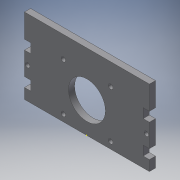
# Autodesk Inventor part: Motor_brace_2
Saved by Autodesk Inventor 2019 (Build 230136000, 136)
## iProperties
Created: 2020-03-11
Part Number: Motor_brace_2
Material: Generic
Document SubType Name: Modeling
Designer: Vijay
Density: 1 g/cm^3
Appearance: Default
Author: Vijay
Autodesk Inventor part; units mm, degrees
ref_plane "YZ Plane" through (0, 0, 0) normal (1, 0, 0) x (0, 1, 0)
ref_plane "XZ Plane" through (0, 0, 0) normal (0, 1, 0) x (-1, 0, 0)
ref_plane "XY Plane" through (0, 0, 0) normal (0, 0, 1) x (1, 0, 0)
sketch "Sketch1" plane through (0, 0, 0) normal (0, 0, 1) x (1, 0, 0)
  line L0 (20, 35.0868) -> (15.0858, 40.001) construction
  line L1 (15.0858, 40.001) -> (-15.0858, 40.001) construction
  line L2 (-15.0858, 40.001) -> (-20, 35.0868) construction
  line L3 (-20, 35.0868) -> (-20, 4.9152) construction
  line L4 (-20, 4.9152) -> (-15.0858, 0.001) construction
  line L5 (-15.0858, 0.001) -> (15.0858, 0.001) construction
  line L6 (15.0858, 0.001) -> (20, 4.9152) construction
  line L7 (20, 4.9152) -> (20, 35.0868) construction
  spline S0 degree 3 poles (-17.5, 4.501) (-17.5, 4.4448) (-17.4976, 4.3891) (-17.4883, 4.2777) (-17.4812, 4.2221) (-17.4625, 4.1117) (-17.4509, 4.0569) (-17.423, 3.9488) (-17.4069, 3.8953) (-17.3846, 3.8313) (-17.3806, 3.8202) (-17.3733, 3.8003) (-17.3701, 3.792) (-17.3645, 3.7774) (-17.3621, 3.7713) (-17.3394, 3.714) (-17.3174, 3.6644) (-17.2693, 3.567) (-17.2432, 3.5192) (-17.1873, 3.4259) (-17.1575, 3.3805) (-17.0943, 3.2923) (-17.061, 3.2495) (-16.9905, 3.1663) (-16.9533, 3.1259) (-16.8745, 3.0471) (-16.8335, 3.0095) (-16.7483, 2.9374) (-16.704, 2.9031) (-16.6129, 2.8383) (-16.566, 2.8079) (-16.4701, 2.7511) (-16.4211, 2.7248) (-16.3422, 2.6867) (-16.3133, 2.6735) (-16.2744, 2.657) (-16.2645, 2.6528) (-16.2484, 2.6463) (-16.2421, 2.6438) (-16.1856, 2.6214) (-16.1347, 2.6037) (-16.0314, 2.5722) (-15.979, 2.5585) (-15.8734, 2.5355) (-15.8202, 2.5261) (-15.7135, 2.5117) (-15.66, 2.5067) (-15.5709, 2.502) (-15.5355, 2.501) (-15.4438, 2.501) (-15.3881, 2.5034) (-15.2767, 2.5127) (-15.2211, 2.5198) (-15.1106, 2.5385) (-15.0559, 2.5501) (-14.9477, 2.578) (-14.8942, 2.5941) (-14.8302, 2.6164) (-14.8192, 2.6204) (-14.7993, 2.6277) (-14.791, 2.6309) (-14.7764, 2.6365) (-14.7703, 2.6389) (-14.713, 2.6616) (-14.6634, 2.6836) (-14.566, 2.7317) (-14.5182, 2.7578) (-14.4249, 2.8137) (-14.3795, 2.8435) (-14.2913, 2.9067) (-14.2485, 2.94) (-14.1653, 3.0105) (-14.1249, 3.0477) (-14.0461, 3.1265) (-14.0085, 3.1675) (-13.9364, 3.2527) (-13.9021, 3.297) (-13.8373, 3.3881) (-13.8069, 3.435) (-13.7501, 3.5309) (-13.7238, 3.5799) (-13.6857, 3.6588) (-13.6725, 3.6877) (-13.656, 3.7265) (-13.6519, 3.7364) (-13.6453, 3.7525) (-13.6428, 3.7589) (-13.6197, 3.8172) (-13.6014, 3.87) (-13.569, 3.9772) (-13.5551, 4.0317) (-13.5319, 4.1414) (-13.5226, 4.1967) (-13.5087, 4.3076) (-13.504, 4.3632) (-13.5006, 4.4464) (-13.5, 4.4736) (-13.5, 4.501) knots 0.5 0.5 0.5 0.5 0.513789 0.513789 0.527784 0.527784 0.541793 0.541793 0.555687 0.555687 0.558594 0.558594 0.560925 0.560925 0.5625 0.5625 0.574861 0.574861 0.587418 0.587418 0.599984 0.599984 0.612492 0.612492 0.625 0.625 0.637686 0.637686 0.650587 0.650587 0.663509 0.663509 0.676325 0.676325 0.683594 0.683594 0.68594 0.68594 0.6875 0.6875 0.700841 0.700841 0.714366 0.714366 0.727891 0.727891 0.741278 0.741278 0.75 0.75 0.76379 0.76379 0.777788 0.777788 0.7918 0.7918 0.805696 0.805696 0.808594 0.808594 0.810925 0.810925 0.8125 0.8125 0.824861 0.824861 0.837418 0.837418 0.849984 0.849984 0.862492 0.862492 0.875 0.875 0.887686 0.887686 0.900587 0.900587 0.913509 0.913509 0.926325 0.926325 0.933594 0.933594 0.935925 0.935925 0.9375 0.9375 0.951347 0.951347 0.96538 0.96538 0.979408 0.979408 0.993282 0.993282 1 1 1 1 construction
  spline S1 degree 3 poles (-13.5, 4.501) (-13.5, 4.5571) (-13.5024, 4.6127) (-13.5117, 4.7238) (-13.5187, 4.7793) (-13.5373, 4.8895) (-13.5489, 4.9441) (-13.5766, 5.0521) (-13.5927, 5.1054) (-13.6151, 5.1697) (-13.6192, 5.1812) (-13.6267, 5.2016) (-13.6299, 5.2101) (-13.6355, 5.2247) (-13.6379, 5.2308) (-13.6606, 5.288) (-13.6826, 5.3376) (-13.7307, 5.435) (-13.7568, 5.4828) (-13.8127, 5.5761) (-13.8425, 5.6215) (-13.9057, 5.7097) (-13.939, 5.7525) (-14.0095, 5.8357) (-14.0467, 5.8761) (-14.1255, 5.9549) (-14.1665, 5.9925) (-14.2517, 6.0646) (-14.296, 6.0989) (-14.3871, 6.1637) (-14.434, 6.1941) (-14.5299, 6.2509) (-14.5789, 6.2772) (-14.6578, 6.3153) (-14.6867, 6.3285) (-14.7256, 6.345) (-14.7355, 6.3492) (-14.7516, 6.3557) (-14.7579, 6.3582) (-14.8144, 6.3806) (-14.8653, 6.3983) (-14.9686, 6.4298) (-15.021, 6.4435) (-15.1266, 6.4665) (-15.1798, 6.4759) (-15.2865, 6.4903) (-15.34, 6.4953) (-15.4291, 6.5) (-15.4645, 6.501) (-15.5562, 6.501) (-15.6119, 6.4986) (-15.7233, 6.4893) (-15.7789, 6.4822) (-15.8894, 6.4635) (-15.9441, 6.4519) (-16.0523, 6.424) (-16.1058, 6.4079) (-16.1698, 6.3856) (-16.1808, 6.3816) (-16.2007, 6.3743) (-16.209, 6.3711) (-16.2236, 6.3655) (-16.2297, 6.3631) (-16.287, 6.3404) (-16.3366, 6.3184) (-16.434, 6.2703) (-16.4818, 6.2442) (-16.5751, 6.1883) (-16.6205, 6.1585) (-16.7087, 6.0953) (-16.7515, 6.062) (-16.8347, 5.9915) (-16.8751, 5.9543) (-16.9539, 5.8755) (-16.9915, 5.8345) (-17.0636, 5.7493) (-17.0979, 5.705) (-17.1627, 5.6139) (-17.1931, 5.567) (-17.2499, 5.4711) (-17.2762, 5.4221) (-17.3143, 5.3432) (-17.3275, 5.3143) (-17.344, 5.2754) (-17.3482, 5.2655) (-17.3547, 5.2494) (-17.3572, 5.2431) (-17.3796, 5.1866) (-17.3973, 5.1357) (-17.4288, 5.0324) (-17.4425, 4.98) (-17.4655, 4.8745) (-17.4749, 4.8213) (-17.4893, 4.7146) (-17.4943, 4.6611) (-17.4991, 4.5719) (-17.5, 4.5366) (-17.5, 4.501) knots 0 0 0 0 0.013787 0.013787 0.027761 0.027761 0.041736 0.041736 0.055579 0.055579 0.058594 0.058594 0.060939 0.060939 0.0625 0.0625 0.074861 0.074861 0.087418 0.087418 0.099984 0.099984 0.112492 0.112492 0.125 0.125 0.137686 0.137686 0.150587 0.150587 0.163509 0.163509 0.176325 0.176325 0.183594 0.183594 0.18594 0.18594 0.1875 0.1875 0.200841 0.200841 0.214366 0.214366 0.227891 0.227891 0.241278 0.241278 0.25 0.25 0.26379 0.26379 0.277788 0.277788 0.2918 0.2918 0.305696 0.305696 0.308594 0.308594 0.310925 0.310925 0.3125 0.3125 0.324861 0.324861 0.337418 0.337418 0.349984 0.349984 0.362492 0.362492 0.375 0.375 0.387686 0.387686 0.400587 0.400587 0.413509 0.413509 0.426325 0.426325 0.433594 0.433594 0.43594 0.43594 0.4375 0.4375 0.450839 0.450839 0.464362 0.464362 0.477886 0.477886 0.49127 0.49127 0.5 0.5 0.5 0.5 construction
  spline S2 degree 3 poles (-17.5, 35.501) (-17.5, 35.4448) (-17.4976, 35.3891) (-17.4883, 35.2777) (-17.4812, 35.2221) (-17.4625, 35.1117) (-17.4509, 35.0569) (-17.423, 34.9488) (-17.4069, 34.8953) (-17.3846, 34.8313) (-17.3806, 34.8202) (-17.3733, 34.8003) (-17.3701, 34.792) (-17.3645, 34.7774) (-17.3621, 34.7713) (-17.3394, 34.714) (-17.3174, 34.6644) (-17.2693, 34.567) (-17.2432, 34.5192) (-17.1873, 34.4259) (-17.1575, 34.3805) (-17.0943, 34.2923) (-17.061, 34.2495) (-16.9905, 34.1663) (-16.9533, 34.1259) (-16.8745, 34.0471) (-16.8335, 34.0095) (-16.7483, 33.9374) (-16.704, 33.9031) (-16.6129, 33.8383) (-16.566, 33.8079) (-16.4701, 33.7511) (-16.4211, 33.7248) (-16.3422, 33.6867) (-16.3133, 33.6735) (-16.2744, 33.657) (-16.2645, 33.6528) (-16.2484, 33.6463) (-16.2421, 33.6438) (-16.1856, 33.6214) (-16.1347, 33.6037) (-16.0314, 33.5722) (-15.979, 33.5585) (-15.8734, 33.5355) (-15.8202, 33.5261) (-15.7135, 33.5117) (-15.66, 33.5067) (-15.5709, 33.502) (-15.5355, 33.501) (-15.4438, 33.501) (-15.3881, 33.5034) (-15.2767, 33.5127) (-15.2211, 33.5198) (-15.1106, 33.5385) (-15.0559, 33.5501) (-14.9477, 33.578) (-14.8942, 33.5941) (-14.8302, 33.6164) (-14.8192, 33.6204) (-14.7993, 33.6277) (-14.791, 33.6309) (-14.7764, 33.6365) (-14.7703, 33.6389) (-14.713, 33.6616) (-14.6634, 33.6836) (-14.566, 33.7317) (-14.5182, 33.7578) (-14.4249, 33.8137) (-14.3795, 33.8435) (-14.2913, 33.9067) (-14.2485, 33.94) (-14.1653, 34.0105) (-14.1249, 34.0477) (-14.0461, 34.1265) (-14.0085, 34.1675) (-13.9364, 34.2527) (-13.9021, 34.297) (-13.8373, 34.3881) (-13.8069, 34.435) (-13.7501, 34.5309) (-13.7238, 34.5799) (-13.6857, 34.6588) (-13.6725, 34.6877) (-13.656, 34.7265) (-13.6519, 34.7364) (-13.6453, 34.7525) (-13.6428, 34.7589) (-13.6197, 34.8172) (-13.6014, 34.87) (-13.569, 34.9772) (-13.5551, 35.0317) (-13.5319, 35.1414) (-13.5226, 35.1967) (-13.5087, 35.3076) (-13.504, 35.3632) (-13.5006, 35.4464) (-13.5, 35.4736) (-13.5, 35.501) knots 0.5 0.5 0.5 0.5 0.513789 0.513789 0.527784 0.527784 0.541793 0.541793 0.555687 0.555687 0.558594 0.558594 0.560925 0.560925 0.5625 0.5625 0.574861 0.574861 0.587418 0.587418 0.599984 0.599984 0.612492 0.612492 0.625 0.625 0.637686 0.637686 0.650587 0.650587 0.663509 0.663509 0.676325 0.676325 0.683594 0.683594 0.68594 0.68594 0.6875 0.6875 0.700841 0.700841 0.714366 0.714366 0.727891 0.727891 0.741278 0.741278 0.75 0.75 0.76379 0.76379 0.777788 0.777788 0.7918 0.7918 0.805696 0.805696 0.808594 0.808594 0.810925 0.810925 0.8125 0.8125 0.824861 0.824861 0.837418 0.837418 0.849984 0.849984 0.862492 0.862492 0.875 0.875 0.887686 0.887686 0.900587 0.900587 0.913509 0.913509 0.926325 0.926325 0.933594 0.933594 0.935925 0.935925 0.9375 0.9375 0.951347 0.951347 0.96538 0.96538 0.979408 0.979408 0.993282 0.993282 1 1 1 1 construction
  spline S3 degree 3 poles (-13.5, 35.501) (-13.5, 35.5571) (-13.5024, 35.6127) (-13.5117, 35.7238) (-13.5187, 35.7793) (-13.5373, 35.8895) (-13.5489, 35.9441) (-13.5766, 36.0521) (-13.5927, 36.1054) (-13.6151, 36.1697) (-13.6192, 36.1812) (-13.6267, 36.2016) (-13.6299, 36.2101) (-13.6355, 36.2247) (-13.6379, 36.2308) (-13.6606, 36.288) (-13.6826, 36.3376) (-13.7307, 36.435) (-13.7568, 36.4828) (-13.8127, 36.5761) (-13.8425, 36.6215) (-13.9057, 36.7097) (-13.939, 36.7525) (-14.0095, 36.8357) (-14.0467, 36.8761) (-14.1255, 36.9549) (-14.1665, 36.9925) (-14.2517, 37.0646) (-14.296, 37.0989) (-14.3871, 37.1637) (-14.434, 37.1941) (-14.5299, 37.2509) (-14.5789, 37.2772) (-14.6578, 37.3153) (-14.6867, 37.3285) (-14.7256, 37.345) (-14.7355, 37.3492) (-14.7516, 37.3557) (-14.7579, 37.3582) (-14.8144, 37.3806) (-14.8653, 37.3983) (-14.9686, 37.4298) (-15.021, 37.4435) (-15.1266, 37.4665) (-15.1798, 37.4759) (-15.2865, 37.4903) (-15.34, 37.4953) (-15.4291, 37.5) (-15.4645, 37.501) (-15.5562, 37.501) (-15.6119, 37.4986) (-15.7233, 37.4893) (-15.7789, 37.4822) (-15.8894, 37.4635) (-15.9441, 37.4519) (-16.0523, 37.424) (-16.1058, 37.4079) (-16.1698, 37.3856) (-16.1808, 37.3816) (-16.2007, 37.3743) (-16.209, 37.3711) (-16.2236, 37.3655) (-16.2297, 37.3631) (-16.287, 37.3404) (-16.3366, 37.3184) (-16.434, 37.2703) (-16.4818, 37.2442) (-16.5751, 37.1883) (-16.6205, 37.1585) (-16.7087, 37.0953) (-16.7515, 37.062) (-16.8347, 36.9915) (-16.8751, 36.9543) (-16.9539, 36.8755) (-16.9915, 36.8345) (-17.0636, 36.7493) (-17.0979, 36.705) (-17.1627, 36.6139) (-17.1931, 36.567) (-17.2499, 36.4711) (-17.2762, 36.4221) (-17.3143, 36.3432) (-17.3275, 36.3143) (-17.344, 36.2754) (-17.3482, 36.2655) (-17.3547, 36.2494) (-17.3572, 36.2431) (-17.3796, 36.1866) (-17.3973, 36.1357) (-17.4288, 36.0324) (-17.4425, 35.98) (-17.4655, 35.8745) (-17.4749, 35.8213) (-17.4893, 35.7146) (-17.4943, 35.6611) (-17.4991, 35.5719) (-17.5, 35.5366) (-17.5, 35.501) knots 0 0 0 0 0.013787 0.013787 0.027761 0.027761 0.041736 0.041736 0.055579 0.055579 0.058594 0.058594 0.060939 0.060939 0.0625 0.0625 0.074861 0.074861 0.087418 0.087418 0.099984 0.099984 0.112492 0.112492 0.125 0.125 0.137686 0.137686 0.150587 0.150587 0.163509 0.163509 0.176325 0.176325 0.183594 0.183594 0.18594 0.18594 0.1875 0.1875 0.200841 0.200841 0.214366 0.214366 0.227891 0.227891 0.241278 0.241278 0.25 0.25 0.26379 0.26379 0.277788 0.277788 0.2918 0.2918 0.305696 0.305696 0.308594 0.308594 0.310925 0.310925 0.3125 0.3125 0.324861 0.324861 0.337418 0.337418 0.349984 0.349984 0.362492 0.362492 0.375 0.375 0.387686 0.387686 0.400587 0.400587 0.413509 0.413509 0.426325 0.426325 0.433594 0.433594 0.43594 0.43594 0.4375 0.4375 0.450839 0.450839 0.464362 0.464362 0.477886 0.477886 0.49127 0.49127 0.5 0.5 0.5 0.5 construction
  circle A0 centre (0, 20.001) radius 11 construction
  spline S4 degree 3 poles (13.5, 35.501) (13.5, 35.4448) (13.5024, 35.3891) (13.5117, 35.2777) (13.5188, 35.2221) (13.5375, 35.1117) (13.5491, 35.0569) (13.577, 34.9488) (13.5931, 34.8953) (13.6154, 34.8313) (13.6194, 34.8202) (13.6267, 34.8003) (13.6299, 34.792) (13.6355, 34.7774) (13.6379, 34.7713) (13.6606, 34.714) (13.6826, 34.6644) (13.7307, 34.567) (13.7568, 34.5192) (13.8127, 34.4259) (13.8425, 34.3805) (13.9057, 34.2923) (13.939, 34.2495) (14.0095, 34.1663) (14.0467, 34.1259) (14.1255, 34.0471) (14.1665, 34.0095) (14.2517, 33.9374) (14.296, 33.9031) (14.3871, 33.8383) (14.434, 33.8079) (14.5299, 33.7511) (14.5789, 33.7248) (14.6578, 33.6867) (14.6867, 33.6735) (14.7256, 33.657) (14.7355, 33.6528) (14.7516, 33.6463) (14.7579, 33.6438) (14.8144, 33.6214) (14.8653, 33.6037) (14.9686, 33.5722) (15.021, 33.5585) (15.1266, 33.5355) (15.1798, 33.5261) (15.2865, 33.5117) (15.34, 33.5067) (15.4291, 33.502) (15.4645, 33.501) (15.5562, 33.501) (15.6119, 33.5034) (15.7233, 33.5127) (15.7789, 33.5198) (15.8894, 33.5385) (15.9441, 33.5501) (16.0523, 33.578) (16.1058, 33.5941) (16.1698, 33.6164) (16.1808, 33.6204) (16.2007, 33.6277) (16.209, 33.6309) (16.2236, 33.6365) (16.2297, 33.6389) (16.287, 33.6616) (16.3366, 33.6836) (16.434, 33.7317) (16.4818, 33.7578) (16.5751, 33.8137) (16.6205, 33.8435) (16.7087, 33.9067) (16.7515, 33.94) (16.8347, 34.0105) (16.8751, 34.0477) (16.9539, 34.1265) (16.9915, 34.1675) (17.0636, 34.2527) (17.0979, 34.297) (17.1627, 34.3881) (17.1931, 34.435) (17.2499, 34.5309) (17.2762, 34.5799) (17.3143, 34.6588) (17.3275, 34.6877) (17.344, 34.7265) (17.3481, 34.7364) (17.3547, 34.7525) (17.3572, 34.7589) (17.3803, 34.8172) (17.3986, 34.87) (17.431, 34.9772) (17.4449, 35.0317) (17.4681, 35.1414) (17.4774, 35.1967) (17.4913, 35.3076) (17.496, 35.3632) (17.4994, 35.4464) (17.5, 35.4736) (17.5, 35.501) knots 0.5 0.5 0.5 0.5 0.513789 0.513789 0.527784 0.527784 0.541793 0.541793 0.555687 0.555687 0.558594 0.558594 0.560925 0.560925 0.5625 0.5625 0.574861 0.574861 0.587418 0.587418 0.599984 0.599984 0.612492 0.612492 0.625 0.625 0.637686 0.637686 0.650587 0.650587 0.663509 0.663509 0.676325 0.676325 0.683594 0.683594 0.68594 0.68594 0.6875 0.6875 0.700841 0.700841 0.714366 0.714366 0.727891 0.727891 0.741278 0.741278 0.75 0.75 0.76379 0.76379 0.777788 0.777788 0.7918 0.7918 0.805696 0.805696 0.808594 0.808594 0.810925 0.810925 0.8125 0.8125 0.824861 0.824861 0.837418 0.837418 0.849984 0.849984 0.862492 0.862492 0.875 0.875 0.887686 0.887686 0.900587 0.900587 0.913509 0.913509 0.926325 0.926325 0.933594 0.933594 0.935925 0.935925 0.9375 0.9375 0.951347 0.951347 0.96538 0.96538 0.979408 0.979408 0.993282 0.993282 1 1 1 1 construction
  spline S5 degree 3 poles (17.5, 35.501) (17.5, 35.5571) (17.4976, 35.6127) (17.4883, 35.7238) (17.4813, 35.7793) (17.4627, 35.8895) (17.4511, 35.9441) (17.4234, 36.0521) (17.4073, 36.1054) (17.3849, 36.1697) (17.3808, 36.1812) (17.3733, 36.2016) (17.3701, 36.2101) (17.3645, 36.2247) (17.3621, 36.2308) (17.3394, 36.288) (17.3174, 36.3376) (17.2693, 36.435) (17.2432, 36.4828) (17.1873, 36.5761) (17.1575, 36.6215) (17.0943, 36.7097) (17.061, 36.7525) (16.9905, 36.8357) (16.9533, 36.8761) (16.8745, 36.9549) (16.8335, 36.9925) (16.7483, 37.0646) (16.704, 37.0989) (16.6129, 37.1637) (16.566, 37.1941) (16.4701, 37.2509) (16.4211, 37.2772) (16.3422, 37.3153) (16.3133, 37.3285) (16.2744, 37.345) (16.2645, 37.3492) (16.2484, 37.3557) (16.2421, 37.3582) (16.1856, 37.3806) (16.1347, 37.3983) (16.0314, 37.4298) (15.979, 37.4435) (15.8734, 37.4665) (15.8202, 37.4759) (15.7135, 37.4903) (15.66, 37.4953) (15.5709, 37.5) (15.5355, 37.501) (15.4438, 37.501) (15.3881, 37.4986) (15.2767, 37.4893) (15.2211, 37.4822) (15.1106, 37.4635) (15.0559, 37.4519) (14.9477, 37.424) (14.8942, 37.4079) (14.8302, 37.3856) (14.8192, 37.3816) (14.7993, 37.3743) (14.791, 37.3711) (14.7764, 37.3655) (14.7703, 37.3631) (14.713, 37.3404) (14.6634, 37.3184) (14.566, 37.2703) (14.5182, 37.2442) (14.4249, 37.1883) (14.3795, 37.1585) (14.2913, 37.0953) (14.2485, 37.062) (14.1653, 36.9915) (14.1249, 36.9543) (14.0461, 36.8755) (14.0085, 36.8345) (13.9364, 36.7493) (13.9021, 36.705) (13.8373, 36.6139) (13.8069, 36.567) (13.7501, 36.4711) (13.7238, 36.4221) (13.6857, 36.3432) (13.6725, 36.3143) (13.656, 36.2754) (13.6518, 36.2655) (13.6453, 36.2494) (13.6428, 36.2431) (13.6204, 36.1866) (13.6027, 36.1357) (13.5712, 36.0324) (13.5575, 35.98) (13.5345, 35.8745) (13.5251, 35.8213) (13.5107, 35.7146) (13.5057, 35.6611) (13.5009, 35.5719) (13.5, 35.5366) (13.5, 35.501) knots 0 0 0 0 0.013787 0.013787 0.027761 0.027761 0.041736 0.041736 0.055579 0.055579 0.058594 0.058594 0.060939 0.060939 0.0625 0.0625 0.074861 0.074861 0.087418 0.087418 0.099984 0.099984 0.112492 0.112492 0.125 0.125 0.137686 0.137686 0.150587 0.150587 0.163509 0.163509 0.176325 0.176325 0.183594 0.183594 0.18594 0.18594 0.1875 0.1875 0.200841 0.200841 0.214366 0.214366 0.227891 0.227891 0.241278 0.241278 0.25 0.25 0.26379 0.26379 0.277788 0.277788 0.2918 0.2918 0.305696 0.305696 0.308594 0.308594 0.310925 0.310925 0.3125 0.3125 0.324861 0.324861 0.337418 0.337418 0.349984 0.349984 0.362492 0.362492 0.375 0.375 0.387686 0.387686 0.400587 0.400587 0.413509 0.413509 0.426325 0.426325 0.433594 0.433594 0.43594 0.43594 0.4375 0.4375 0.450839 0.450839 0.464362 0.464362 0.477886 0.477886 0.49127 0.49127 0.5 0.5 0.5 0.5 construction
  spline S6 degree 3 poles (13.5, 4.501) (13.5, 4.4448) (13.5024, 4.3891) (13.5117, 4.2777) (13.5188, 4.2221) (13.5375, 4.1117) (13.5491, 4.0569) (13.577, 3.9488) (13.5931, 3.8953) (13.6154, 3.8313) (13.6194, 3.8202) (13.6267, 3.8003) (13.6299, 3.792) (13.6355, 3.7774) (13.6379, 3.7713) (13.6606, 3.714) (13.6826, 3.6644) (13.7307, 3.567) (13.7568, 3.5192) (13.8127, 3.4259) (13.8425, 3.3805) (13.9057, 3.2923) (13.939, 3.2495) (14.0095, 3.1663) (14.0467, 3.1259) (14.1255, 3.0471) (14.1665, 3.0095) (14.2517, 2.9374) (14.296, 2.9031) (14.3871, 2.8383) (14.434, 2.8079) (14.5299, 2.7511) (14.5789, 2.7248) (14.6578, 2.6867) (14.6867, 2.6735) (14.7256, 2.657) (14.7355, 2.6528) (14.7516, 2.6463) (14.7579, 2.6438) (14.8144, 2.6214) (14.8653, 2.6037) (14.9686, 2.5722) (15.021, 2.5585) (15.1266, 2.5355) (15.1798, 2.5261) (15.2865, 2.5117) (15.34, 2.5067) (15.4291, 2.502) (15.4645, 2.501) (15.5562, 2.501) (15.6119, 2.5034) (15.7233, 2.5127) (15.7789, 2.5198) (15.8894, 2.5385) (15.9441, 2.5501) (16.0523, 2.578) (16.1058, 2.5941) (16.1698, 2.6164) (16.1808, 2.6204) (16.2007, 2.6277) (16.209, 2.6309) (16.2236, 2.6365) (16.2297, 2.6389) (16.287, 2.6616) (16.3366, 2.6836) (16.434, 2.7317) (16.4818, 2.7578) (16.5751, 2.8137) (16.6205, 2.8435) (16.7087, 2.9067) (16.7515, 2.94) (16.8347, 3.0105) (16.8751, 3.0477) (16.9539, 3.1265) (16.9915, 3.1675) (17.0636, 3.2527) (17.0979, 3.297) (17.1627, 3.3881) (17.1931, 3.435) (17.2499, 3.5309) (17.2762, 3.5799) (17.3143, 3.6588) (17.3275, 3.6877) (17.344, 3.7265) (17.3481, 3.7364) (17.3547, 3.7525) (17.3572, 3.7589) (17.3803, 3.8172) (17.3986, 3.87) (17.431, 3.9772) (17.4449, 4.0317) (17.4681, 4.1414) (17.4774, 4.1967) (17.4913, 4.3076) (17.496, 4.3632) (17.4994, 4.4464) (17.5, 4.4736) (17.5, 4.501) knots 0.5 0.5 0.5 0.5 0.513789 0.513789 0.527784 0.527784 0.541793 0.541793 0.555687 0.555687 0.558594 0.558594 0.560925 0.560925 0.5625 0.5625 0.574861 0.574861 0.587418 0.587418 0.599984 0.599984 0.612492 0.612492 0.625 0.625 0.637686 0.637686 0.650587 0.650587 0.663509 0.663509 0.676325 0.676325 0.683594 0.683594 0.68594 0.68594 0.6875 0.6875 0.700841 0.700841 0.714366 0.714366 0.727891 0.727891 0.741278 0.741278 0.75 0.75 0.76379 0.76379 0.777788 0.777788 0.7918 0.7918 0.805696 0.805696 0.808594 0.808594 0.810925 0.810925 0.8125 0.8125 0.824861 0.824861 0.837418 0.837418 0.849984 0.849984 0.862492 0.862492 0.875 0.875 0.887686 0.887686 0.900587 0.900587 0.913509 0.913509 0.926325 0.926325 0.933594 0.933594 0.935925 0.935925 0.9375 0.9375 0.951347 0.951347 0.96538 0.96538 0.979408 0.979408 0.993282 0.993282 1 1 1 1 construction
  spline S7 degree 3 poles (17.5, 4.501) (17.5, 4.5571) (17.4976, 4.6127) (17.4883, 4.7238) (17.4813, 4.7793) (17.4627, 4.8895) (17.4511, 4.9441) (17.4234, 5.0521) (17.4073, 5.1054) (17.3849, 5.1697) (17.3808, 5.1812) (17.3733, 5.2016) (17.3701, 5.2101) (17.3645, 5.2247) (17.3621, 5.2308) (17.3394, 5.288) (17.3174, 5.3376) (17.2693, 5.435) (17.2432, 5.4828) (17.1873, 5.5761) (17.1575, 5.6215) (17.0943, 5.7097) (17.061, 5.7525) (16.9905, 5.8357) (16.9533, 5.8761) (16.8745, 5.9549) (16.8335, 5.9925) (16.7483, 6.0646) (16.704, 6.0989) (16.6129, 6.1637) (16.566, 6.1941) (16.4701, 6.2509) (16.4211, 6.2772) (16.3422, 6.3153) (16.3133, 6.3285) (16.2744, 6.345) (16.2645, 6.3492) (16.2484, 6.3557) (16.2421, 6.3582) (16.1856, 6.3806) (16.1347, 6.3983) (16.0314, 6.4298) (15.979, 6.4435) (15.8734, 6.4665) (15.8202, 6.4759) (15.7135, 6.4903) (15.66, 6.4953) (15.5709, 6.5) (15.5355, 6.501) (15.4438, 6.501) (15.3881, 6.4986) (15.2767, 6.4893) (15.2211, 6.4822) (15.1106, 6.4635) (15.0559, 6.4519) (14.9477, 6.424) (14.8942, 6.4079) (14.8302, 6.3856) (14.8192, 6.3816) (14.7993, 6.3743) (14.791, 6.3711) (14.7764, 6.3655) (14.7703, 6.3631) (14.713, 6.3404) (14.6634, 6.3184) (14.566, 6.2703) (14.5182, 6.2442) (14.4249, 6.1883) (14.3795, 6.1585) (14.2913, 6.0953) (14.2485, 6.062) (14.1653, 5.9915) (14.1249, 5.9543) (14.0461, 5.8755) (14.0085, 5.8345) (13.9364, 5.7493) (13.9021, 5.705) (13.8373, 5.6139) (13.8069, 5.567) (13.7501, 5.4711) (13.7238, 5.4221) (13.6857, 5.3432) (13.6725, 5.3143) (13.656, 5.2754) (13.6518, 5.2655) (13.6453, 5.2494) (13.6428, 5.2431) (13.6204, 5.1866) (13.6027, 5.1357) (13.5712, 5.0324) (13.5575, 4.98) (13.5345, 4.8745) (13.5251, 4.8213) (13.5107, 4.7146) (13.5057, 4.6611) (13.5009, 4.5719) (13.5, 4.5366) (13.5, 4.501) knots 0 0 0 0 0.013787 0.013787 0.027761 0.027761 0.041736 0.041736 0.055579 0.055579 0.058594 0.058594 0.060939 0.060939 0.0625 0.0625 0.074861 0.074861 0.087418 0.087418 0.099984 0.099984 0.112492 0.112492 0.125 0.125 0.137686 0.137686 0.150587 0.150587 0.163509 0.163509 0.176325 0.176325 0.183594 0.183594 0.18594 0.18594 0.1875 0.1875 0.200841 0.200841 0.214366 0.214366 0.227891 0.227891 0.241278 0.241278 0.25 0.25 0.26379 0.26379 0.277788 0.277788 0.2918 0.2918 0.305696 0.305696 0.308594 0.308594 0.310925 0.310925 0.3125 0.3125 0.324861 0.324861 0.337418 0.337418 0.349984 0.349984 0.362492 0.362492 0.375 0.375 0.387686 0.387686 0.400587 0.400587 0.413509 0.413509 0.426325 0.426325 0.433594 0.433594 0.43594 0.43594 0.4375 0.4375 0.450839 0.450839 0.464362 0.464362 0.477886 0.477886 0.49127 0.49127 0.5 0.5 0.5 0.5 construction
  line L8 (-152.3368, 49.5885) -> (152.3133, 49.5884) construction
  line L9 (-40.8871, 0.001) -> (40.8871, 0.001)
  line L10 (40.8871, 0.001) -> (40.8871, 40.001)
  line L11 (40.8871, 40.001) -> (-40.8871, 40.001)
  line L12 (-40.8871, 40.001) -> (-40.8871, 0.001)
  line L13 (-40.8871, 0.001) -> (40.8871, 40.001) construction
  line L14 (40.8871, 0.001) -> (-40.8871, 40.001) construction
  line L15 (40.8871, 40.001) -> (-40.8871, 40.001)
  line L16 (-40.8871, 40.001) -> (-40.8871, 49.5885)
  line L17 (-40.8871, 49.5885) -> (40.8871, 49.5885)
  line L18 (40.8871, 49.5885) -> (40.8871, 40.001)
  circle A1 centre (15.5, 4.501) radius 1.5 projected
  circle A2 centre (-15.5, 4.501) radius 1.5 projected
  circle A3 centre (-15.5, 35.501) radius 1.5 projected
  circle A4 centre (15.5, 35.501) radius 1.5 projected
  circle A5 centre (0, 20.001) radius 12.0934
  point P0 (0, 0)
  constraints: 20 end point, 4 parallel, 2 horizontal, 2 midpoint, 2 perpendicular, 1 centre point, 1 coincident, 1 point on line
extrude "Extrusion1" add sketch "Sketch1" along normal blind 4
sketch "Sketch2" plane through (0, 0, 4) normal (0, 0, 1) x (1, 0, 0)
  line L0 (36.8871, 28.0768) -> (36.8871, 34.0768) construction
  line L1 (36.8871, 28.0768) -> (40.8871, 28.0768) construction
  line L2 (40.8871, 34.0768) -> (40.8871, 28.0768) construction
  line L3 (36.8871, 34.0768) -> (40.8871, 34.0768) construction
  line L4 (36.8871, 6.8768) -> (36.8871, 12.8768) construction
  line L5 (36.8871, 6.8768) -> (40.8871, 6.8768) construction
  line L6 (40.8871, 12.8768) -> (40.8871, 6.8768) construction
  line L7 (36.8871, 12.8768) -> (40.8871, 12.8768) construction
  line L8 (-40.8871, 28.0768) -> (-40.8871, 34.0768) construction
  line L9 (-40.8871, 28.0768) -> (-36.8871, 28.0768) construction
  line L10 (-36.8871, 34.0768) -> (-36.8871, 28.0768) construction
  line L11 (-40.8871, 34.0768) -> (-36.8871, 34.0768) construction
  line L12 (-40.8871, 6.8768) -> (-40.8871, 12.8768) construction
  line L13 (-40.8871, 6.8768) -> (-36.8871, 6.8768) construction
  line L14 (-36.8871, 12.8768) -> (-36.8871, 6.8768) construction
  line L15 (-40.8871, 12.8768) -> (-36.8871, 12.8768) construction
  line L16 (-40.8871, 18.9768) -> (-40.8871, 21.9768) construction
  line L17 (-40.8871, 18.9768) -> (-36.8871, 18.9768) construction
  line L18 (-36.8871, 21.9768) -> (-36.8871, 18.9768) construction
  line L19 (-40.8871, 21.9768) -> (-36.8871, 21.9768) construction
  line L20 (36.8871, 18.9768) -> (36.8871, 21.9768) construction
  line L21 (36.8871, 18.9768) -> (40.8871, 18.9768) construction
  line L22 (40.8871, 21.9768) -> (40.8871, 18.9768) construction
  line L23 (36.8871, 21.9768) -> (40.8871, 21.9768) construction
  circle A0 centre (-38.8871, 20.4768) radius 1.6
  circle A1 centre (38.8871, 20.4768) radius 1.6
  line L24 (-36.6871, 34.2768) -> (-36.6871, 27.8768)
  line L25 (-36.6871, 27.8768) -> (-41.0871, 27.8768)
  line L26 (-41.0871, 27.8768) -> (-41.0871, 34.2768)
  line L27 (-41.0871, 34.2768) -> (-36.6871, 34.2768)
  line L28 (-36.6871, 13.0768) -> (-36.6871, 6.6768)
  line L29 (-36.6871, 6.6768) -> (-41.0871, 6.6768)
  line L30 (-41.0871, 6.6768) -> (-41.0871, 13.0768)
  line L31 (-41.0871, 13.0768) -> (-36.6871, 13.0768)
  line L32 (41.0871, 34.2768) -> (41.0871, 27.8768)
  line L33 (41.0871, 27.8768) -> (36.6871, 27.8768)
  line L34 (36.6871, 27.8768) -> (36.6871, 34.2768)
  line L35 (36.6871, 34.2768) -> (41.0871, 34.2768)
  line L36 (41.0871, 13.0768) -> (41.0871, 6.6768)
  line L37 (41.0871, 6.6768) -> (36.6871, 6.6768)
  line L38 (36.6871, 6.6768) -> (36.6871, 13.0768)
  line L39 (36.6871, 13.0768) -> (41.0871, 13.0768)
  point P0 (0, 0)
  dimension "d2" = 3.2
  dimension "d3" = 3.2
  dimension "d4" = 0.2
  dimension "d5" = 0.2
  dimension "d6" = 0.2
  dimension "d7" = 0.2
  constraints: 32 end point, 2 centre point, 12 other
  measures "d2" diameter of A0
  measures "d3" diameter of A1
  measures "d4" distance between parallel lines of L11 L27
  measures "d5" distance between parallel lines of L15 L31
  measures "d6" distance between parallel lines of L3 L35
  measures "d7" distance between parallel lines of L7 L39
extrude "Extrusion2" cut sketch "Sketch2" against normal through all
sketch "Sketch3" plane through (0, 0, 4) normal (0, 0, 1) x (1, 0, 0)
  point P0 (0, 0)
body "Solid1"
